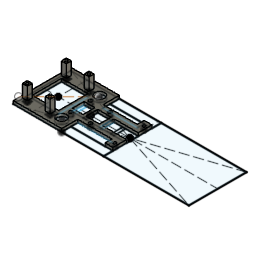
baseMount (Autodesk Fusion 360 design; units mm, degrees)
Autodesk Fusion 360 part; units mm, degrees
sketch "Sketch1" plane through (0, 0, 0) normal (0, 0, 1) x (1, 0, 0)
  line L0 (90, 29.5) -> (-90, 29.5)
  line L1 (-90, 29.5) -> (-90, -29.5)
  line L2 (-90, -29.5) -> (90, -29.5)
  line L3 (90, -29.5) -> (90, 29.5)
  line L4 (90, 29.5) -> (-90, -29.5) construction
  line L5 (-90, 29.5) -> (90, -29.5) construction
  line L6 (-40.35, 29.5) -> (-40.35, -29.5) construction
  line L7 (-82.5, 17.5) -> (-87.5, 17.5)
  line L8 (-87.5, 17.5) -> (-87.5, 22.5)
  line L9 (-87.5, 22.5) -> (-82.5, 22.5)
  line L10 (-82.5, 22.5) -> (-82.5, 17.5)
  line L11 (-82.5, 17.5) -> (-87.5, 22.5) construction
  line L12 (-87.5, 17.5) -> (-82.5, 22.5) construction
  line L13 (-90, 0) -> (90, 0) construction
  line L14 (-87.5, -22.5) -> (-82.5, -22.5)
  line L15 (-87.5, -17.5) -> (-87.5, -22.5)
  line L16 (-82.5, -22.5) -> (-82.5, -17.5)
  line L17 (-82.5, -17.5) -> (-87.5, -17.5)
  line L18 (-73.35, 29.5) -> (-73.35, -29.5) construction
  line L19 (-64.2, 22.5) -> (-64.2, 17.5)
  line L20 (-59.2, 17.5) -> (-59.2, 22.5)
  line L21 (-59.2, 22.5) -> (-64.2, 22.5)
  line L22 (-64.2, 17.5) -> (-59.2, 17.5)
  line L23 (-59.2, -17.5) -> (-59.2, -22.5)
  line L24 (-64.2, -22.5) -> (-64.2, -17.5)
  line L25 (-59.2, -22.5) -> (-64.2, -22.5)
  line L26 (-64.2, -17.5) -> (-59.2, -17.5)
  circle A0 centre (-50.35, 10) radius 1.8
  circle A1 centre (-50.35, -10) radius 1.8
  circle A2 centre (-30.35, 10) radius 1.8
  circle A3 centre (-30.35, -10) radius 1.8
  circle A4 centre (-0.35, 15) radius 1.5
  circle A5 centre (-0.35, -15) radius 1.5
  line L27 (90, 29.5) -> (2.65, 29.5)
  line L28 (2.65, 29.5) -> (2.65, -29.5)
  line L29 (2.65, -29.5) -> (90, -29.5)
  line L30 (90, -29.5) -> (90, 29.5)
  circle A6 centre (-85, 20) radius 1.3
  circle A7 centre (-85, -20) radius 1.3
  circle A8 centre (-61.7, 20) radius 1.3
  circle A9 centre (-61.7, -20) radius 1.3
  line L31 (-93.8102, -20.3) -> (-52.8898, 20.3) construction
  line L32 (2.65, -6) -> (-52.8898, -6)
  line L33 (-52.8898, -6) -> (-52.8898, 6)
  line L34 (-52.8898, 6) -> (2.65, 6)
  line L35 (2.65, 6) -> (2.65, -6)
  line L36 (-0.35, 15) -> (-0.35, 29.5) construction
  line L37 (-40.35, 29.5) -> (2.65, 29.5)
  line L38 (2.65, 29.5) -> (2.65, 20)
  line L39 (2.65, 20) -> (-40.35, 20)
  line L40 (-40.35, 20) -> (-40.35, 29.5)
  line L41 (2.65, -20) -> (-40.35, -20)
  line L42 (-40.35, -20) -> (-40.35, -29.5)
  line L43 (-40.35, -29.5) -> (2.65, -29.5)
  line L44 (2.65, -29.5) -> (2.65, -20)
  line L45 (-25.1199, 6) -> (-22.1199, 6)
  line L46 (-22.1199, 6) -> (-22.1199, -6)
  line L47 (-22.1199, -6) -> (-25.1199, -6)
  line L48 (-25.1199, -6) -> (-25.1199, 6)
  line L49 (-13.35, 6) -> (-10.35, 6)
  line L50 (-10.35, 6) -> (-10.35, -6)
  line L51 (-10.35, -6) -> (-13.35, -6)
  line L52 (-13.35, -6) -> (-13.35, 6)
  line L53 (-40.35, -20) -> (-5.35, -20)
  line L54 (-5.35, -20) -> (-5.35, -13)
  line L55 (-5.35, -13) -> (-40.35, -13)
  line L56 (-40.35, -13) -> (-40.35, -20)
  line L57 (-40.35, 20) -> (-5.35, 20)
  line L58 (-5.35, 20) -> (-5.35, 13)
  line L59 (-5.35, 13) -> (-40.35, 13)
  line L60 (-40.35, 13) -> (-40.35, 20)
  line L61 (-52.8898, 6) -> (-49.8898, 6)
  line L62 (-49.8898, 6) -> (-49.8898, -6)
  line L63 (-49.8898, -6) -> (-52.8898, -6)
  line L64 (-52.8898, -6) -> (-52.8898, 6)
  line L65 (-57.8898, -15) -> (-85, -15)
  line L66 (-85, -15) -> (-85, 15)
  line L67 (-85, 15) -> (-57.8898, 15)
  line L68 (-57.8898, 15) -> (-57.8898, -15)
  circle A10 centre (-50.35, 19.5) radius 5
  circle A11 centre (-50.35, -19.5) radius 5
  line L69 (-38.85, -6) -> (-41.85, -6)
  line L70 (-41.85, -6) -> (-41.85, 6)
  line L71 (-41.85, 6) -> (-38.85, 6)
  line L72 (-38.85, 6) -> (-38.85, -6)
  line L73 (-38.85, -6) -> (-41.85, 6) construction
  line L74 (-41.85, -6) -> (-38.85, 6) construction
  point P0 (-85, 20)
  point P1 (-85, -20)
  point P2 (-61.7, 20)
  point P3 (-61.7, -20)
  point P4 (-85, -20)
  point P5 (-73.35, 0)
  point P6 (-40.35, 0)
  point P7 (-40.35, 0)
  dimension "batteryPillarWidth" = 5
  dimension "batteryPillarLength" = 5
  dimension "d4" = 33
  dimension "d5" = 11.65
  dimension "baseLength" = 180
  dimension "flightcontrolScrew" = 3.6
  dimension "d8" = 10
  dimension "d9" = 10
  dimension "opticalflowScrew" = 3
  dimension "d11" = 40
  dimension "opticalFlowDistance" = 15
  dimension "d13" = 3
  dimension "d14" = 2.6
  dimension "d17" = 5
  dimension "d23" = 4
  dimension "d24" = 4
  dimension "d25" = 5
  dimension "d26" = 3
  dimension "d27" = 3
  dimension "d28" = 10
  dimension "d30" = 5
  dimension "d31" = 3
  dimension "d34" = 5
  dimension "d35" = 5
  dimension "d36" = 2.5
  dimension "d37" = 20
  dimension "d38" = 10
  dimension "d39" = 10
  dimension "d40" = 10
  dimension "d43" = 3
  dimension "d48" = 7
  dimension "d50" = 30
  constraint horizontal L0
  constraint perpendicular L0 L1
  constraint parallel L0 L2
  constraint parallel L1 L3
  constraint coincident L4 origin
  constraint coincident L5 origin
  constraint horizontal L7
  constraint perpendicular L7 L8
  constraint parallel L7 L9
  constraint parallel L8 L10
  constraint coincident L11 P0
  constraint coincident L12 P0
  constraint midpoint L1 L13.start
  constraint midpoint L3 L13.end
  constraint symmetric L7.start L13 L16.end
  constraint symmetric L7.end L13 L15.start
  constraint symmetric L8.end L13 L14.start
  constraint symmetric L9.end L13 L14.end
  constraint symmetric P0 L13 P4
  constraint coincident L0 L18.start
  constraint coincident L2 L18.end
  constraint perpendicular L2 L18
  constraint symmetric L7.start L18 L19.end
  constraint symmetric L7.end L18 L20.start
  constraint symmetric L8.end L18 L20.end
  constraint symmetric L9.end L18 L19.start
  constraint symmetric P0 L18 P2
  constraint symmetric L13 P2 P3
  constraint symmetric L13 L19.start L24.start
  constraint symmetric L13 L19.end L24.end
  constraint symmetric L13 L20.start L23.start
  constraint symmetric L13 L20.end L23.end
  constraint symmetric L13 A0 A1
  constraint symmetric L6 A0 A2
  constraint symmetric L6 A1 A3
  constraint symmetric L13 A4 A5
  constraint horizontal L27
  constraint vertical L28
  constraint horizontal L29
  constraint vertical L30
  constraint coincident L2 L28.end
  constraint coincident P0 A6.centre
  constraint symmetric L13 A6 A7
  constraint symmetric L18 A6 A8
  constraint symmetric L18 A7 A9
  constraint coincident L31 P5
  constraint midpoint L18 P5
  constraint midpoint L6 P7
  constraint horizontal L32
  constraint vertical L33
  constraint horizontal L34
  constraint vertical L35
  constraint coincident L28 L32.start
  constraint coincident A4.centre L36.start
  constraint coincident L0 L36.end
  constraint perpendicular L0 L36
  constraint horizontal L37
  constraint vertical L38
  constraint horizontal L39
  constraint vertical L40
  constraint coincident L28 L38.end
  constraint symmetric L6.start L13 L6.end
  constraint symmetric L13 L27.end L28.end
  constraint symmetric L13 L38.end L41.start
  constraint symmetric L13 L39.end L41.end
  constraint horizontal L45
  constraint vertical L46
  constraint horizontal L47
  constraint vertical L48
  constraint midpoint L34 L45.start
  constraint horizontal L49
  constraint vertical L50
  constraint horizontal L51
  constraint vertical L52
  constraint coincident L34 L49.start
  constraint horizontal L53
  constraint vertical L54
  constraint horizontal L55
  constraint vertical L56
  constraint symmetric L13 L41.end L39.end
  constraint symmetric L13 L53.end L57.end
  constraint symmetric L13 L54.end L58.end
  constraint symmetric L13 L55.end L59.end
  constraint horizontal L61
  constraint vertical L62
  constraint horizontal L63
  constraint vertical L64
  constraint coincident L32 L62.end
  constraint horizontal L65
  constraint vertical L66
  constraint horizontal L67
  constraint vertical L68
  constraint symmetric L13 A10 A11
  constraint horizontal L69
  constraint perpendicular L69 L70
  constraint parallel L69 L71
  constraint parallel L70 L72
  constraint coincident L32 L69.start
  constraint coincident L73 P7
  constraint coincident L74 P7
  constraint coincident P7 P6
  constraint collinear L2 L43
  constraint collinear L32 L47
  constraint collinear L32 L51
  constraint collinear L34 L71
  measures "batteryPillarWidth" distance of L8.end L9.end
  measures "batteryPillarLength" distance of L7.end L8.end
  measures "d4" distance of L6 L18
  measures "d5" distance of P0 L18
  measures "baseLength" distance of L1 L3
  measures "flightcontrolScrew" diameter of A0
  measures "d8" distance of L13 A0.centre
  measures "d9" distance of L6 A0.centre
  measures "opticalflowScrew" diameter of A4
  measures "d11" distance of L6 A4.centre
  measures "opticalFlowDistance" distance of L13 A4.centre
  measures "d13" distance of A4.centre L28
  measures "d14" diameter of A6
  measures "d17" distance of L1 P0
  measures "d23" distance of A0.centre L34
  measures "d24" distance of A3.centre L32
  measures "d25" distance of A4.centre L39
  measures "d26" distance of L45.start L45.end
  measures "d27" distance of L49.start L49.end
  measures "d28" distance of L36 L50
  measures "d30" distance of A5.centre L54
  measures "d31" distance of L33.end L61.end
  measures "d34" distance of L1 L66
  measures "d35" distance of L64 L68
  measures "d36" distance of L26 L65
  measures "d37" distance of P0 L13
  measures "d38" diameter of A10
  measures "d39" distance of L0 A10.centre
  measures "d40" distance of L6 A10.centre
  measures "d43" distance of L70 L72
  measures "d48" distance of L2 L14
  measures "d50" distance of L65 L67
extrude "Extrude10" add sketch "Sketch1" along normal blind 3 contours L0 L1 L2 L28 L32 L33 L34 L39 L40 L41 L42 L45 L47 L49 L51 L54 L55 L56 L58 L59 L60 L61 L63 L64 L69 L71 | L32 L34 L45 L46 L47 L48 | L32 L34 L69 L70 L71 L72
extrude "Extrude11" add sketch "Sketch1" along normal blind 16 contours L7 L8 L9 L10 | L14 L15 L16 L17 | L19 L20 L21 L22 | L23 L24 L25 L26
extrude "Extrude8" [suppressed]
extrude "Extrude9" [suppressed]
extrude "Extrude6" [suppressed]
extrude "Extrude7" [suppressed]
extrude "Extrude5" [suppressed]
extrude "Extrude4" [suppressed]
extrude "Extrude3" [suppressed]
extrude "Extrude2" [suppressed]
